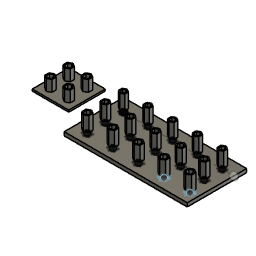
Conduit entretoise et écrou v9 (Autodesk Fusion 360 design; units mm, degrees)
Autodesk Fusion 360 part; units mm, degrees
sketch "Esquisse1" plane through (0, 0, 0) normal (0, 1, 0) x (1, 0, 0)
  line L0 (-2.25, 1.299) -> (-2.25, -1.299)
  line L1 (-2.25, -1.299) -> (0, -2.5981)
  line L2 (0, -2.5981) -> (2.25, -1.299)
  line L3 (2.25, -1.299) -> (2.25, 1.299)
  line L4 (2.25, 1.299) -> (0, 2.5981)
  line L5 (0, 2.5981) -> (-2.25, 1.299)
  line L6 (-3.45, 1.9919) -> (-3.45, -1.9919)
  line L7 (-3.45, -1.9919) -> (0, -3.9837)
  line L8 (0, -3.9837) -> (3.45, -1.9919)
  line L9 (3.45, -1.9919) -> (3.45, 1.9919)
  line L10 (3.45, 1.9919) -> (0, 3.9837)
  line L11 (0, 3.9837) -> (-3.45, 1.9919)
  line L12 (29.25, 1.3279) -> (26.95, 2.6558)
  line L13 (24.65, -1.3279) -> (26.95, -2.6558)
  line L14 (26.95, -4.0415) -> (30.45, -2.0207)
  line L15 (29.25, -1.3279) -> (29.25, 1.3279)
  line L16 (24.65, 1.3279) -> (24.65, -1.3279)
  line L17 (30.45, -2.0207) -> (30.45, 2.0207)
  line L18 (26.95, 4.0415) -> (23.45, 2.0207)
  line L19 (26.95, 2.6558) -> (24.65, 1.3279)
  line L20 (23.45, -2.0207) -> (26.95, -4.0415)
  line L21 (23.45, 2.0207) -> (23.45, -2.0207)
  line L22 (26.95, -2.6558) -> (29.25, -1.3279)
  line L23 (30.45, 2.0207) -> (26.95, 4.0415)
  line L24 (56.35, 1.3568) -> (54, 2.7135)
  line L25 (51.65, -1.3568) -> (54, -2.7135)
  line L26 (54, -4.0992) -> (57.55, -2.0496)
  line L27 (56.35, -1.3568) -> (56.35, 1.3568)
  line L28 (51.65, 1.3568) -> (51.65, -1.3568)
  line L29 (57.55, -2.0496) -> (57.55, 2.0496)
  line L30 (54, 4.0992) -> (50.45, 2.0496)
  line L31 (54, 2.7135) -> (51.65, 1.3568)
  line L32 (50.45, -2.0496) -> (54, -4.0992)
  line L33 (50.45, 2.0496) -> (50.45, -2.0496)
  line L34 (54, -2.7135) -> (56.35, -1.3568)
  line L35 (57.55, 2.0496) -> (54, 4.0992)
  line L36 (83.55, 1.3856) -> (81.15, 2.7713)
  line L37 (78.75, -1.3856) -> (81.15, -2.7713)
  line L38 (81.15, -4.1569) -> (84.75, -2.0785)
  line L39 (83.55, -1.3856) -> (83.55, 1.3856)
  line L40 (78.75, 1.3856) -> (78.75, -1.3856)
  line L41 (84.75, -2.0785) -> (84.75, 2.0785)
  line L42 (81.15, 4.1569) -> (77.55, 2.0785)
  line L43 (81.15, 2.7713) -> (78.75, 1.3856)
  line L44 (77.55, -2.0785) -> (81.15, -4.1569)
  line L45 (77.55, 2.0785) -> (77.55, -2.0785)
  line L46 (81.15, -2.7713) -> (83.55, -1.3856)
  line L47 (84.75, 2.0785) -> (81.15, 4.1569)
  line L48 (2.25, 1.299) -> (0, 2.5981)
  line L49 (-2.25, -1.299) -> (0, -2.5981)
  line L50 (0, -3.9837) -> (3.45, -1.9919)
  line L51 (2.25, -1.299) -> (2.25, 1.299)
  line L52 (-2.25, 1.299) -> (-2.25, -1.299)
  line L53 (3.45, -1.9919) -> (3.45, 1.9919)
  line L54 (0, 3.9837) -> (-3.45, 1.9919)
  line L55 (0, 2.5981) -> (-2.25, 1.299)
  line L56 (-3.45, -1.9919) -> (0, -3.9837)
  line L57 (-3.45, 1.9919) -> (-3.45, -1.9919)
  line L58 (0, -2.5981) -> (2.25, -1.299)
  line L59 (3.45, 1.9919) -> (0, 3.9837)
  line L60 (110.85, 1.4145) -> (108.4, 2.829)
  line L61 (105.95, -1.4145) -> (108.4, -2.829)
  line L62 (108.4, -4.2147) -> (112.05, -2.1073)
  line L63 (110.85, -1.4145) -> (110.85, 1.4145)
  line L64 (105.95, 1.4145) -> (105.95, -1.4145)
  line L65 (112.05, -2.1073) -> (112.05, 2.1073)
  line L66 (108.4, 4.2147) -> (104.75, 2.1073)
  line L67 (108.4, 2.829) -> (105.95, 1.4145)
  line L68 (104.75, -2.1073) -> (108.4, -4.2147)
  line L69 (104.75, 2.1073) -> (104.75, -2.1073)
  line L70 (108.4, -2.829) -> (110.85, -1.4145)
  line L71 (112.05, 2.1073) -> (108.4, 4.2147)
  line L72 (2.75, -18.5566) -> (0.25, -17.1132)
  line L73 (-2.25, -21.4434) -> (0.25, -22.8868)
  line L74 (0.25, -24.2724) -> (3.95, -22.1362)
  line L75 (2.75, -21.4434) -> (2.75, -18.5566)
  line L76 (-2.25, -18.5566) -> (-2.25, -21.4434)
  line L77 (3.95, -22.1362) -> (3.95, -17.8638)
  line L78 (0.25, -15.7276) -> (-3.45, -17.8638)
  line L79 (0.25, -17.1132) -> (-2.25, -18.5566)
  line L80 (-3.45, -22.1362) -> (0.25, -24.2724)
  line L81 (-3.45, -17.8638) -> (-3.45, -22.1362)
  line L82 (0.25, -22.8868) -> (2.75, -21.4434)
  line L83 (3.95, -17.8638) -> (0.25, -15.7276)
  line L84 (30.25, -18.5278) -> (27.7, -17.0555)
  line L85 (25.15, -21.4722) -> (27.7, -22.9445)
  line L86 (27.7, -24.3301) -> (31.45, -22.1651)
  line L87 (30.25, -21.4722) -> (30.25, -18.5278)
  line L88 (25.15, -18.5278) -> (25.15, -21.4722)
  line L89 (31.45, -22.1651) -> (31.45, -17.8349)
  line L90 (27.7, -15.6699) -> (23.95, -17.8349)
  line L91 (27.7, -17.0555) -> (25.15, -18.5278)
  line L92 (23.95, -22.1651) -> (27.7, -24.3301)
  line L93 (23.95, -17.8349) -> (23.95, -22.1651)
  line L94 (27.7, -22.9445) -> (30.25, -21.4722)
  line L95 (31.45, -17.8349) -> (27.7, -15.6699)
  line L96 (57.85, -18.4989) -> (55.25, -16.9978)
  line L97 (52.65, -21.5011) -> (55.25, -23.0022)
  line L98 (55.25, -24.3879) -> (59.05, -22.1939)
  line L99 (57.85, -21.5011) -> (57.85, -18.4989)
  line L100 (52.65, -18.4989) -> (52.65, -21.5011)
  line L101 (59.05, -22.1939) -> (59.05, -17.8061)
  line L102 (55.25, -15.6121) -> (51.45, -17.8061)
  line L103 (55.25, -16.9978) -> (52.65, -18.4989)
  line L104 (51.45, -22.1939) -> (55.25, -24.3879)
  line L105 (51.45, -17.8061) -> (51.45, -22.1939)
  line L106 (55.25, -23.0022) -> (57.85, -21.5011)
  line L107 (59.05, -17.8061) -> (55.25, -15.6121)
  line L108 (111.35, -18.4412) -> (108.65, -16.8823)
  line L109 (105.95, -21.5588) -> (108.65, -23.1177)
  line L110 (108.65, -24.5033) -> (112.55, -22.2517)
  line L111 (111.35, -21.5588) -> (111.35, -18.4412)
  line L112 (105.95, -18.4412) -> (105.95, -21.5588)
  line L113 (112.55, -22.2517) -> (112.55, -17.7483)
  line L114 (108.65, -15.4967) -> (104.75, -17.7483)
  line L115 (108.65, -16.8823) -> (105.95, -18.4412)
  line L116 (104.75, -22.2517) -> (108.65, -24.5033)
  line L117 (104.75, -17.7483) -> (104.75, -22.2517)
  line L118 (108.65, -23.1177) -> (111.35, -21.5588)
  line L119 (112.55, -17.7483) -> (108.65, -15.4967)
  line L120 (31.25, -38.3834) -> (28.45, -36.7668)
  line L121 (28.45, -43.2332) -> (31.25, -41.6166)
  line L122 (56.5, -35.3235) -> (52.45, -37.6617)
  line L123 (32.45, -37.6906) -> (28.45, -35.3812)
  line L124 (31.25, -41.6166) -> (31.25, -38.3834)
  line L125 (28.45, -35.3812) -> (24.45, -37.6906)
  line L126 (24.45, -42.3094) -> (28.45, -44.6188)
  line L127 (28.45, -36.7668) -> (25.65, -38.3834)
  line L128 (24.45, -37.6906) -> (24.45, -42.3094)
  line L129 (86.75, -22.2228) -> (86.75, -17.7772)
  line L130 (-3.45, -37.7195) -> (-3.45, -42.2805)
  line L131 (79.05, -17.7772) -> (79.05, -22.2228)
  line L132 (82.9, -23.06) -> (85.55, -21.53)
  line L133 (3.25, -41.5877) -> (3.25, -38.4123)
  line L134 (80.25, -18.47) -> (80.25, -21.53)
  line L135 (85.55, -21.53) -> (85.55, -18.47)
  line L136 (0.5, -36.8246) -> (-2.25, -38.4123)
  line L137 (-2.25, -38.4123) -> (-2.25, -41.5877)
  line L138 (25.65, -41.6166) -> (28.45, -43.2332)
  line L139 (86.75, -17.7772) -> (82.9, -15.5544)
  line L140 (82.9, -24.4456) -> (86.75, -22.2228)
  line L141 (85.55, -18.47) -> (82.9, -16.94)
  line L142 (-2.25, -41.5877) -> (0.5, -43.1754)
  line L143 (25.65, -38.3834) -> (25.65, -41.6166)
  line L144 (4.45, -42.2805) -> (4.45, -37.7195)
  line L145 (82.9, -16.94) -> (80.25, -18.47)
  line L146 (0.5, -35.4389) -> (-3.45, -37.7195)
  line L147 (80.25, -21.53) -> (82.9, -23.06)
  line L148 (79.05, -22.2228) -> (82.9, -24.4456)
  line L149 (32.45, -42.3094) -> (32.45, -37.6906)
  line L150 (56.5, -43.2909) -> (59.35, -41.6454)
  line L151 (53.65, -38.3546) -> (53.65, -41.6454)
  line L152 (56.5, -36.7091) -> (53.65, -38.3546)
  line L153 (52.45, -42.3383) -> (56.5, -44.6765)
  line L154 (52.45, -37.6617) -> (52.45, -42.3383)
  line L155 (53.65, -41.6454) -> (56.5, -43.2909)
  line L156 (59.35, -38.3546) -> (56.5, -36.7091)
  line L157 (59.35, -41.6454) -> (59.35, -38.3546)
  line L158 (28.45, -44.6188) -> (32.45, -42.3094)
  line L159 (0.5, -44.5611) -> (4.45, -42.2805)
  line L160 (117.05, -37.604) -> (112.9, -35.208)
  line L161 (4.45, -37.7195) -> (0.5, -35.4389)
  line L162 (108.75, -42.396) -> (112.9, -44.792)
  line L163 (0.5, -43.1754) -> (3.25, -41.5877)
  line L164 (82.9, -15.5544) -> (79.05, -17.7772)
  line L165 (115.85, -41.7032) -> (115.85, -38.2968)
  line L166 (3.25, -38.4123) -> (0.5, -36.8246)
  line L167 (56.5, -44.6765) -> (60.55, -42.3383)
  line L168 (112.9, -35.208) -> (108.75, -37.604)
  line L169 (112.9, -44.792) -> (117.05, -42.396)
  line L170 (-3.45, -42.2805) -> (0.5, -44.5611)
  line L171 (117.05, -42.396) -> (117.05, -37.604)
  line L172 (60.55, -42.3383) -> (60.55, -37.6617)
  line L173 (60.55, -37.6617) -> (56.5, -35.3235)
  line L174 (109.95, -41.7032) -> (112.9, -43.4064)
  line L175 (109.95, -38.2968) -> (109.95, -41.7032)
  line L176 (112.9, -43.4064) -> (115.85, -41.7032)
  line L177 (115.85, -38.2968) -> (112.9, -36.5936)
  line L178 (112.9, -36.5936) -> (109.95, -38.2968)
  line L179 (108.75, -37.604) -> (108.75, -42.396)
  line L180 (0, 0) -> (121, 0) construction
  line L181 (87.4, -38.3257) -> (84.5, -36.6514)
  line L182 (80.4, -42.3671) -> (84.5, -44.7343)
  line L183 (88.6, -37.6329) -> (84.5, -35.2657)
  line L184 (84.5, -44.7343) -> (88.6, -42.3671)
  line L185 (84.5, -43.3486) -> (87.4, -41.6743)
  line L186 (84.5, -36.6514) -> (81.6, -38.3257)
  line L187 (84.5, -35.2657) -> (80.4, -37.6329)
  line L188 (81.6, -41.6743) -> (84.5, -43.3486)
  line L189 (80.4, -37.6329) -> (80.4, -42.3671)
  line L190 (81.6, -38.3257) -> (81.6, -41.6743)
  line L191 (88.6, -42.3671) -> (88.6, -37.6329)
  line L192 (87.4, -41.6743) -> (87.4, -38.3257)
  point P0 (26.95, 0)
  point P1 (26.95, 0)
  point P2 (26.95, 0)
  point P3 (54, 0)
  point P4 (54, 0)
  point P5 (54, 0)
  point P6 (81.15, 0)
  point P7 (81.15, 0)
  point P8 (81.15, 0)
  point P9 (108.4, 0)
  point P10 (108.4, 0)
  point P11 (108.4, 0)
  point P12 (0.25, -20)
  point P13 (0.25, -20)
  point P14 (0.25, -20)
  point P15 (27.7, -20)
  point P16 (27.7, -20)
  point P17 (27.7, -20)
  point P18 (55.25, -20)
  point P19 (55.25, -20)
  point P20 (55.25, -20)
  point P21 (108.65, -20)
  point P22 (108.65, -20)
  point P23 (108.65, -20)
  point P24 (56.5, -40)
  point P25 (56.5, -40)
  point P26 (112.9, -40)
  point P27 (112.9, -40)
  point P28 (56.5, -40)
  point P29 (0.5, -40)
  point P30 (0.5, -40)
  point P31 (0.5, -40)
  point P32 (112.9, -40)
  point P33 (28.45, -40)
  point P34 (28.45, -40)
  point P35 (28.45, -40)
  point P36 (82.9, -20)
  point P37 (82.9, -20)
  point P38 (82.9, -20)
  point P39 (84.5, -40)
  point P40 (84.5, -40)
  point P41 (84.5, -40)
  dimension "d4" = 1.2
  dimension "d5" = 4.5
  dimension "d6" = 1.2
  dimension "d7" = 4.6
  dimension "d8" = 1.2
  dimension "d9" = 4.7
  dimension "d10" = 1.2
  dimension "d11" = 4.8
  dimension "d12" = 1.2
  dimension "d13" = 4.5
  dimension "d14" = 1.2
  dimension "d15" = 4.9
  dimension "d18" = 1.2
  dimension "d19" = 5
  dimension "d20" = 1.2
  dimension "d21" = 5.1
  dimension "d22" = 1.2
  dimension "d23" = 5.2
  dimension "d26" = 1.2
  dimension "d27" = 5.4
  dimension "d28" = 1.2
  dimension "d29" = 5.5
  dimension "d30" = 1.2
  dimension "d31" = 5.6
  dimension "d32" = 1.2
  dimension "d33" = 5.7
  dimension "d34" = 1.2
  dimension "d35" = 5.3
  dimension "d36" = 1.2
  dimension "d37" = 5.9
  dimension "d40" = 20
  dimension "d41" = 20
  dimension "d42" = 20
  dimension "d44" = 20
  dimension "d47" = 20
  dimension "d48" = 20
  dimension "d51" = 20
  dimension "d52" = 20
  dimension "d54" = 20
  dimension "d55" = 20
  dimension "d56" = 20
  dimension "d57" = 20
  dimension "d58" = 20
  dimension "d60" = 20
  dimension "d61" = 20
  dimension "d62" = 20
  dimension "d63" = 20
  dimension "d64" = 18
  dimension "d65" = 1.2
  dimension "d66" = 5.8
  dimension "d68" = 20
  dimension "d69" = 20.15
  constraint parallel L3 L9
  constraint coincident L180.start origin
  constraint vertical L6
  constraint parallel L15 L17
  constraint coincident P2 P1
  constraint vertical L21
  constraint parallel L27 L29
  constraint coincident P5 P4
  constraint vertical L33
  constraint parallel L39 L41
  constraint coincident P8 P7
  constraint vertical L45
  constraint parallel L51 L53
  constraint vertical L57
  constraint parallel L63 L65
  constraint coincident P11 P10
  constraint vertical L69
  constraint parallel L75 L77
  constraint coincident P14 P13
  constraint vertical L81
  constraint parallel L87 L89
  constraint coincident P17 P16
  constraint vertical L93
  constraint parallel L99 L101
  constraint coincident P20 P19
  constraint vertical L105
  constraint parallel L111 L113
  constraint coincident P23 P22
  constraint vertical L117
  constraint parallel L133 L144
  constraint coincident P31 P30
  constraint vertical L130
  constraint parallel L124 L149
  constraint coincident P35 P34
  constraint vertical L128
  constraint parallel L157 L172
  constraint coincident P28 P25
  constraint vertical L154
  constraint parallel L129 L135
  constraint coincident P38 P37
  constraint vertical L131
  constraint parallel L165 L171
  constraint coincident P32 P27
  constraint vertical L179
  constraint collinear L6 L81
  constraint collinear L6 L130
  constraint perpendicular L64 L180
  constraint coincident P2 L180
  constraint coincident P5 L180
  constraint coincident P8 L180
  constraint coincident P11 L180
  constraint parallel L191 L192
  constraint coincident P41 P40
  constraint vertical L189
  measures "d4" distance of L0 L6
  measures "d5" distance of L0 L3
  measures "d6" distance of L16 L21
  measures "d7" distance of L15 L16
  measures "d8" distance of L28 L33
  measures "d9" distance of L27 L28
  measures "d10" distance of L40 L45
  measures "d11" distance of L39 L40
  measures "d12" distance of L52 L57
  measures "d13" distance of L51 L52
  measures "d14" distance of L64 L69
  measures "d15" distance of L63 L64
  measures "d18" distance of L76 L81
  measures "d19" distance of L75 L76
  measures "d20" distance of L88 L93
  measures "d21" distance of L87 L88
  measures "d22" distance of L100 L105
  measures "d23" distance of L99 L100
  measures "d26" distance of L112 L117
  measures "d27" distance of L111 L112
  measures "d28" distance of L130 L137
  measures "d29" distance of L133 L137
  measures "d30" distance of L128 L143
  measures "d31" distance of L124 L143
  measures "d32" distance of L151 L154
  measures "d33" distance of L151 L157
  measures "d34" distance of L131 L134
  measures "d35" distance of L134 L135
  measures "d36" distance of L175 L179
  measures "d37" distance of L165 L175
  measures "d40" distance of L9 L21
  measures "d41" distance of L41 L69
  measures "d42" distance of L29 L45
  measures "d44" distance of L17 L33
  measures "d47" distance of L89 L105
  measures "d48" distance of L77 L93
  measures "d51" distance of L149 L154
  measures "d52" distance of L128 L144
  measures "d54" vertical distance of L180.start P14
  measures "d55" vertical distance of P14 P31
  measures "d56" vertical distance of P2 P16
  measures "d57" vertical distance of P17 P35
  measures "d58" vertical distance of P5 P20
  measures "d60" vertical distance of P20 P28
  measures "d61" vertical distance of P23 P32
  measures "d62" vertical distance of P11 P23
  measures "d63" vertical distance of P8 P38
  measures "d64" distance of L117 L129
  measures "d65" distance of L189 L190
  measures "d66" distance of L190 L192
  measures "d68" distance of L101 L131
  measures "d69" distance of L179 L191
extrude "Extrusion1" add sketch "Esquisse1" along normal blind 20 contours L6 L7 L8 L9 L10 L11 L50 L53 L54 L56 L57 L59 | L14 L17 L18 L20 L21 L23 | L26 L29 L30 L32 L33 L35 | L38 L41 L42 L44 L45 L47 | L62 L65 L66 L68 L69 L71 | L74 L77 L78 L80 L81 L83 | L86 L89 L90 L92 L93 L95 | L98 L101 L102 L104 L105 L107 | L110 L113 L114 L116 L117 L119 | L122 L153 L154 L167 L172 L173 | L123 L125 L126 L128 L149 L158 | L129 L131 L139 L140 L148 L164 | L130 L144 L146 L159 L161 L170 | L160 L162 L168 L169 L171 L179 makes body 1 at (51.6333, 6.6667, 2.7328) makes body 2 at (53.8, 6.6667, 43.1177) makes body 3 at (1.4833, 13.3333, 16.4397) makes body 4 at (31.1167, 6.6667, 36.9208) makes body 5 at (106.05, 6.6667, 23.0022) makes body 6 at (28.1167, 6.6667, 3.3679) makes body 7 at (78.75, 13.3333, 2.7713) makes body 8 at (59.05, 6.6667, 20.7313) makes body 9 at (84.1833, 6.6667, 23.7047) makes body 10 at (1.15, 13.3333, 3.3198) makes body 11 at (-3.45, 6.6667, 39.2398) makes body 12 at (111.5167, 6.6667, 36.0067) makes body 13 at (30.2, 13.3333, 17.1132) makes body 14 at (110.8333, 13.3333, -2.8098)
extrude "Extrusion2" add sketch "Esquisse1" along normal blind 20 separate body contours L182 L183 L184 L187 L189 L191 makes body 15
sketch "Esquisse2" plane through (0, 0, 0) normal (0, 1, 0) x (1, 0, 0)
  line L0 (-10, 10) -> (125, 10)
  line L1 (125, 10) -> (125, -55)
  line L2 (125, -55) -> (-10, -55)
  line L3 (-10, -55) -> (-10, 10)
  constraint horizontal L0
  constraint vertical L1
  constraint horizontal L2
  constraint vertical L3
extrude "Extrusion3" add sketch "Esquisse2" along normal blind 4 bodies 1 5 4 3 2 8 7 6 12 11 10 9 13 14 15
sketch "Esquisse3" plane through (0, 0, 0) normal (0, 1, 0) x (1, 0, 0)
  line L0 (-70, 10) -> (-30, 10)
  line L1 (-30, 10) -> (-30, -30)
  line L2 (-30, -30) -> (-70, -30)
  line L3 (-70, -30) -> (-70, 10)
  line L4 (-62.8, 1.6166) -> (-62.8, -1.6166)
  line L5 (-62.8, -1.6166) -> (-60, -3.2332)
  line L6 (-60, -3.2332) -> (-57.2, -1.6166)
  line L7 (-57.2, -1.6166) -> (-57.2, 1.6166)
  line L8 (-57.2, 1.6166) -> (-60, 3.2332)
  line L9 (-60, 3.2332) -> (-62.8, 1.6166)
  line L10 (-64, 2.3094) -> (-64, -2.3094)
  line L11 (-64, -2.3094) -> (-60, -4.6188)
  line L12 (-60, -4.6188) -> (-56, -2.3094)
  line L13 (-56, -2.3094) -> (-56, 2.3094)
  line L14 (-56, 2.3094) -> (-60, 4.6188)
  line L15 (-60, 4.6188) -> (-64, 2.3094)
  line L16 (-10, 10) -> (-10, -55)
  line L17 (125, 10) -> (-10, 10)
  line L18 (-40, -3.2332) -> (-37.2, -1.6166)
  line L19 (-42.8, -1.6166) -> (-40, -3.2332)
  line L20 (-42.8, 1.6166) -> (-42.8, -1.6166)
  line L21 (-44, 2.3094) -> (-44, -2.3094)
  line L22 (-36, 2.3094) -> (-40, 4.6188)
  line L23 (-37.2, 1.6166) -> (-40, 3.2332)
  line L24 (-44, -2.3094) -> (-40, -4.6188)
  line L25 (-40, 4.6188) -> (-44, 2.3094)
  line L26 (-40, 3.2332) -> (-42.8, 1.6166)
  line L27 (-40, -4.6188) -> (-36, -2.3094)
  line L28 (-36, -2.3094) -> (-36, 2.3094)
  line L29 (-37.2, -1.6166) -> (-37.2, 1.6166)
  line L30 (-56, -17.6906) -> (-60, -15.3812)
  line L31 (-62.8, -21.6166) -> (-60, -23.2332)
  line L32 (-56, -22.3094) -> (-56, -17.6906)
  line L33 (-60, -24.6188) -> (-56, -22.3094)
  line L34 (-60, -15.3812) -> (-64, -17.6906)
  line L35 (-62.8, -18.3834) -> (-62.8, -21.6166)
  line L36 (-57.2, -21.6166) -> (-57.2, -18.3834)
  line L37 (-60, -23.2332) -> (-57.2, -21.6166)
  line L38 (-57.2, -18.3834) -> (-60, -16.7668)
  line L39 (-60, -16.7668) -> (-62.8, -18.3834)
  line L40 (-64, -22.3094) -> (-60, -24.6188)
  line L41 (-64, -17.6906) -> (-64, -22.3094)
  line L42 (-36, -22.3094) -> (-36, -17.6906)
  line L43 (-44, -17.6906) -> (-44, -22.3094)
  line L44 (-40, -23.2332) -> (-37.2, -21.6166)
  line L45 (-42.8, -21.6166) -> (-40, -23.2332)
  line L46 (-37.2, -18.3834) -> (-40, -16.7668)
  line L47 (-40, -16.7668) -> (-42.8, -18.3834)
  line L48 (-42.8, -18.3834) -> (-42.8, -21.6166)
  line L49 (-44, -22.3094) -> (-40, -24.6188)
  line L50 (-36, -17.6906) -> (-40, -15.3812)
  line L51 (-40, -15.3812) -> (-44, -17.6906)
  line L52 (-40, -24.6188) -> (-36, -22.3094)
  line L53 (-37.2, -21.6166) -> (-37.2, -18.3834)
  point P0 (-60, 0)
  point P1 (-60, 0)
  point P2 (-40, 0)
  point P3 (-40, 0)
  point P4 (-60, -20)
  point P5 (-60, -20)
  point P6 (-40, -20)
  point P7 (-40, -20)
  dimension "d76" = 5.6
  dimension "d80" = 1.2
  dimension "d81" = 40
  dimension "d82" = 40
  dimension "d83" = 10
  dimension "d85" = 10
  dimension "d86" = 20
  dimension "d87" = 5.6
  dimension "d88" = 1.2
  dimension "d89" = 5.6
  dimension "d90" = 1.2
  dimension "d91" = 5.6
  dimension "d92" = 1.2
  dimension "d93" = 10
  dimension "d94" = 10
  dimension "d95" = 10
  dimension "d96" = 10
  dimension "d97" = 10
  dimension "d98" = 10
  constraint horizontal L0
  constraint vertical L1
  constraint horizontal L2
  constraint vertical L3
  constraint vertical L7
  constraint vertical L13
  constraint coincident P1 P0
  constraint collinear L0 L17
  constraint vertical L29
  constraint vertical L28
  constraint coincident P3 P2
  constraint vertical L36
  constraint vertical L32
  constraint coincident P5 P4
  constraint vertical L53
  constraint vertical L42
  constraint coincident P7 P6
  measures "d76" distance of L4 L7
  measures "d80" distance of L7 L13
  measures "d81" distance of L0.start L0.end
  measures "d82" distance of L0.end L1.end
  measures "d83" distance of L0 P1
  measures "d85" distance of L3 P1
  measures "d86" distance of L1 L16
  measures "d87" distance of L20 L29
  measures "d88" distance of L28 L29
  measures "d89" distance of L35 L36
  measures "d90" distance of L32 L36
  measures "d91" distance of L48 L53
  measures "d92" distance of L42 L53
  measures "d93" distance of L3 P5
  measures "d94" distance of L2 P5
  measures "d95" distance of L2 P7
  measures "d96" distance of L1 P7
  measures "d97" distance of L1 P3
  measures "d98" distance of L0 P3
extrude "Extrusion6" add sketch "Esquisse3" along normal blind 2 separate body contours L0 L1 L2 L3 | L4 L5 L6 L7 L8 L9 | L10 L11 L12 L13 L14 L15 | L18 L19 L20 L23 L26 L29 | L21 L22 L24 L25 L27 L28 | L30 L32 L33 L34 L40 L41 | L31 L35 L36 L37 L38 L39 | L42 L43 L49 L50 L51 L52 | L44 L45 L46 L47 L48 L53 makes body 16
extrude "Extrusion7" add sketch "Esquisse3" along normal blind 14.2 contours L10 L11 L12 L13 L14 L15 | L21 L22 L24 L25 L27 L28 | L30 L32 L33 L34 L40 L41 | L42 L43 L49 L50 L51 L52 bodies 16
equation "Ext_entretoise = 4.5 mm"
equation "Ext_ecrou = 5.3 mm"
equation "Epaisseur = 1.2 mm"
equation "d4 = Epaisseur"
equation "d5 = Ext_entretoise"
equation "d6 = Epaisseur"
equation "d7 = Ext_entretoise + 0.1 mm"
equation "d8 = Epaisseur"
equation "d9 = Ext_entretoise + 0.2 mm"
equation "d10 = Epaisseur"
equation "d11 = Ext_entretoise + 0.3 mm"
equation "d12 = Epaisseur"
equation "d13 = Ext_entretoise"
equation "d14 = Epaisseur"
equation "d15 = Ext_entretoise + 0.4 mm"
equation "d18 = Epaisseur"
equation "d19 = Ext_entretoise + 0.5 mm"
equation "d20 = Epaisseur"
equation "d21 = Ext_entretoise + 0.6 mm"
equation "d22 = Epaisseur"
equation "d23 = Ext_entretoise + 0.7 mm"
equation "d26 = Epaisseur"
equation "d27 = Ext_entretoise + 0.9 mm"
equation "d28 = Epaisseur"
equation "d29 = Ext_entretoise + 1 mm"
equation "d30 = Epaisseur"
equation "d31 = Ext_entretoise + 1.1 mm"
equation "d32 = Epaisseur"
equation "d33 = Ext_entretoise + 1.2 mm"
equation "d34 = Epaisseur"
equation "d35 = Ext_entretoise + 0.8 mm"
equation "d36 = Epaisseur"
equation "d37 = Ext_entretoise + 1.4 mm"
equation "d40 = Ecart"
equation "d41 = Ecart"
equation "d42 = Ecart"
equation "Ecart = 20 mm"
equation "d44 = Ecart"
equation "d47 = Ecart"
equation "d48 = Ecart"
equation "d51 = Ecart"
equation "d52 = Ecart"
equation "d54 = Ecart"
equation "d55 = Ecart"
equation "d56 = Ecart"
equation "d57 = Ecart"
equation "d58 = Ecart"
equation "d60 = Ecart"
equation "d61 = Ecart"
equation "d62 = Ecart"
equation "d63 = Ecart"
equation "d65 = Epaisseur"
equation "d66 = Ext_entretoise + 1.3 mm"
equation "d68 = Ecart"
equation "H_ecrou = 2.2 mm"
equation "H_entretoise = 10 mm"
equation "d76 = ecrou"
equation "ecrou = 5.6 mm"
equation "entretoise = 4.9 mm"
equation "d80 = Epaisseur"
equation "d87 = ecrou"
equation "d88 = Epaisseur"
equation "d89 = ecrou"
equation "d90 = Epaisseur"
equation "d91 = ecrou"
equation "d92 = Epaisseur"
equation "d105 = 2 mm + H_ecrou + H_entretoise"
